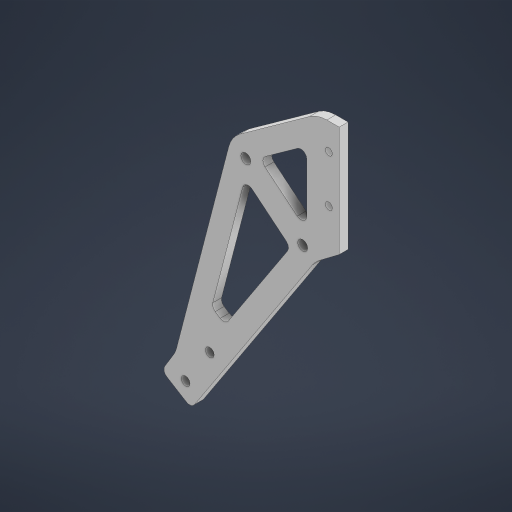
# Autodesk Inventor part: Tibia
Saved by Autodesk Inventor 2024 (Build 280153000, 153)
## iProperties
Created: 2024-06-02
Part Number: Tibia
Material: Generic
Document SubType Name: Modeling
Designer: Hemant
Density: 1 g/cm^3
Appearance: Default
Author: Hemant
Autodesk Inventor part; units mm, degrees
ref_plane "YZ Plane" through (0, 0, 0) normal (1, 0, 0) x (0, 1, 0)
ref_plane "XZ Plane" through (0, 0, 0) normal (0, 1, 0) x (-1, 0, 0)
ref_plane "XY Plane" through (0, 0, 0) normal (0, 0, 1) x (1, 0, 0)
sketch "Sketch1" plane through (0, 0, 0) normal (0, 0, 1) x (1, 0, 0)
  circle A0 centre (-10.7682, 28.6531) radius 1.7
  line L0 (-30.9487, -53.1184) -> (-37.6576, -49.0166)
  arc A1 (-38.3208, -46.2671) -> (-37.6576, -49.0166) centre (-36.6144, -47.3103) ccw
  line L1 (-38.3208, -46.2671) -> (-35.4427, -41.5596)
  arc A2 (-35.4427, -41.5596) -> (-34.2964, -38.8601) centre (-43.9745, -36.3434) ccw
  line L2 (-34.2964, -38.8601) -> (-16.5771, 29.2821)
  arc A3 (-12.739, 34.883) -> (-16.5771, 29.2821) centre (-6.899, 26.7655) ccw
  line L3 (-12.739, 34.883) -> (10.9377, 51.9167)
  arc A4 (16.7777, 53.7992) -> (10.9377, 51.9167) centre (16.7777, 43.7992) ccw
  line L4 (16.7777, 53.7992) -> (20.9818, 53.7992)
  line L5 (20.9818, 45.9992) -> (20.9818, 16.274)
  line L6 (20.9818, 16.274) -> (14.228, 11.1802)
  arc A5 (14.228, 11.1802) -> (11.8867, 8.6795) centre (20.2494, 3.1963) ccw
  line L7 (11.8867, 8.6795) -> (-28.2329, -52.5086)
  arc A6 (-4.1413, 32.6124) -> (-4.2418, 29.4427) centre (-2.9733, 30.9889) ccw
  line L8 (-4.2418, 29.4427) -> (6.7132, 20.4547)
  arc A7 (6.7132, 20.4547) -> (9.9818, 22.0009) centre (7.9818, 22.0009) ccw
  line L9 (9.9818, 22.0009) -> (9.9818, 38.8703)
  arc A8 (9.9818, 38.8703) -> (6.8138, 40.4938) centre (7.9818, 38.8703) ccw
  line L10 (6.8138, 40.4938) -> (-4.1413, 32.6124)
  circle A9 centre (17.4818, 44.7992) radius 1.2
  circle A10 centre (17.4818, 28.7992) radius 1.2
  line L11 (-16.6946, -22.1449) -> (3.4303, 8.5485)
  arc A11 (3.4303, 8.5485) -> (3.0263, 11.1914) centre (1.7578, 9.6452) ccw
  line L12 (3.0263, 11.1914) -> (-8.6289, 20.7539)
  arc A12 (-8.6289, 20.7539) -> (-11.8331, 19.711) centre (-9.8975, 19.2077) ccw
  line L13 (-11.8331, 19.711) -> (-22.01, -19.4256)
  arc A13 (-22.01, -19.4256) -> (-21.171, -21.6014) centre (-20.0743, -19.9289) ccw
  line L14 (-21.171, -21.6014) -> (-19.4638, -22.7208)
  arc A14 (-19.4638, -22.7208) -> (-16.6946, -22.1449) centre (-18.3672, -21.0482) ccw
  line L15 (20.9818, 45.9992) -> (20.9818, 53.7992)
  circle A15 centre (-31.2454, -47.0794) radius 1.5
  circle A16 centre (-23.0206, -34.5354) radius 1.5
  line L16 (-23.0206, -34.5354) -> (-31.2454, -47.0794) construction
  line L17 (-31.2454, -47.0794) -> (-33.987, -51.2608) construction
  arc A17 (-30.9487, -53.1184) -> (-28.2329, -52.5086) centre (-29.9054, -51.412) ccw
  circle A18 centre (8.5593, 12.796) radius 1.7
  line L18 (-10.7682, 28.6531) -> (8.5593, 12.796) construction
  point P0 (0, 0)
  point P1 (-30.3165, -53.5049)
  point P2 (-11.731, -27.3408)
  dimension "d2" = 3
  dimension "d3" = 3
  dimension "d5" = 2
  dimension "d6" = 5
  dimension "d7" = 15
  dimension "d8" = 3.4
  dimension "d9" = 25
  constraints: 38 end point, 26 point on circle, 19 centre point, 3 point on line, 2 parallel, 2 tangent, 1 collinear, 1 perpendicular, 1 other
  measures "d2" diameter of A15
  measures "d3" diameter of A16
  measures "d5" radius of A17
  measures "d6" distance of L16.end L17.end
  measures "d7" distance of L16.start L16.end
  measures "d8" diameter of A18
  measures "d9" distance of L18.start L18.end
extrude "Extrusion1" add sketch "Sketch1" along normal blind 3
body "Solid1"
